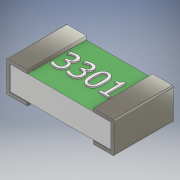
# Autodesk Inventor part: 21-1001
Saved by Autodesk Inventor 2018 (Build 220112000, 112)
## iProperties
Created: 2019-09-21
Part Number: 21-1001
Material: Copper
Document SubType Name: Modeling
Designer: Bradley
Density: 8.94 g/cm^3
Appearance: Smooth - White
Author: Bradley
Autodesk Inventor part; units mm, degrees
ref_plane "YZ Plane" through (0, 0, 0) normal (1, 0, 0) x (0, 1, 0)
ref_plane "XZ Plane" through (0, 0, 0) normal (0, 1, 0) x (-1, 0, 0)
ref_plane "XY Plane" through (0, 0, 0) normal (0, 0, 1) x (1, 0, 0)
sketch "Sketch1" plane through (0, 0, 0) normal (0, 1, 0) x (-1, 0, 0)
  line L0 (0.725, 0.175) -> (-0.725, 0.175)
  line L1 (-0.725, 0.175) -> (-0.725, -0.175)
  line L2 (-0.725, -0.175) -> (0.725, -0.175)
  line L3 (0.725, -0.175) -> (0.725, 0.175)
  line L4 (0.475, 0.175) -> (0.475, 0.225)
  line L5 (0.475, 0.225) -> (0.775, 0.225)
  line L6 (0.775, 0.225) -> (0.775, -0.225)
  line L7 (0.775, -0.225) -> (0.475, -0.225)
  line L8 (0.475, -0.225) -> (0.475, -0.175)
  line L9 (-0.475, 0.175) -> (-0.475, 0.225)
  line L10 (-0.475, 0.225) -> (-0.775, 0.225)
  line L11 (-0.775, 0.225) -> (-0.775, -0.225)
  line L12 (-0.775, -0.225) -> (-0.475, -0.225)
  line L13 (-0.475, -0.175) -> (-0.475, -0.225)
  line L14 (0.475, 0.175) -> (-0.475, 0.175)
  point P0 (0, 0)
  point P1 (0, 0.175)
  point P2 (0.725, 0)
  dimension "d0" = 1.55
  dimension "d1" = 0.05
  dimension "d2" = 0.05
  dimension "d3" = 0.45
  dimension "d4" = 0.3
  constraints: 30 end point, 12 point on line, 7 perpendicular, 3 collinear, 3 midpoint, 2 parallel, 1 horizontal, 1 horizontal alignment, 1 vertical, 1 vertical alignment
  measures "d0" distance between parallel lines of L11 L6
  measures "d1" distance of L7.end L8.end
  measures "d2" distance between parallel lines of L6 L3
  measures "d3" distance of L5.end L6.end
  measures "d4" distance of L6.end L7.end
extrude "Extrusion1" add sketch "Sketch1" along normal mid plane 0.85 contours L0 L4 L5 L6 L7 L8 L2 L3 | L0 L1 L2 L13 L12 L11 L10 L9
extrude "Extrusion2" add sketch "Sketch1" along normal mid plane 0.84 contours L3 L2 L1 L0
sketch "Sketch2" plane through (-0.475, -0.42, 0.175) normal (0, 0, 1) x (1, 0, 0)
  line L0 (0, 0) -> (0, 0.84) projected
  line L1 (0.95, 0) -> (0, 0) projected
  line L2 (0.95, 0) -> (0.95, 0.84) projected
  line L3 (0, 0.84) -> (0.95, 0.84) projected
  line L4 (0, 0.42) -> (0.95, 0.42) construction
  spline S0 degree 2 poles (0.1276, 0.5416) (0.1167, 0.5416) (0.095, 0.5362) (0.0846, 0.5321) knots 0 0 0 1 2 2 2
  spline S1 degree 2 poles (0.0846, 0.5321) (0.0748, 0.5279) (0.0605, 0.5192) (0.0549, 0.5153) knots 0 0 0 1 2 2 2
  line L5 (0.0549, 0.5153) -> (0.0525, 0.5153)
  line L6 (0.0525, 0.5153) -> (0.0525, 0.5578)
  spline S2 degree 2 poles (0.0525, 0.5578) (0.0656, 0.5649) (0.1106, 0.5763) (0.1308, 0.5763) knots 0 0 0 1 2 2 2
  spline S3 degree 2 poles (0.1308, 0.5763) (0.1512, 0.5763) (0.1816, 0.5681) (0.194, 0.5593) knots 0 0 0 1 2 2 2
  spline S4 degree 2 poles (0.194, 0.5593) (0.2071, 0.5498) (0.2207, 0.5224) (0.2207, 0.5039) knots 0 0 0 1 2 2 2
  spline S5 degree 2 poles (0.2207, 0.5039) (0.2207, 0.4791) (0.1881, 0.4416) (0.1653, 0.4368) knots 0 0 0 1 2 2 2
  line L7 (0.1653, 0.4368) -> (0.1653, 0.4339)
  spline S6 degree 2 poles (0.1653, 0.4339) (0.1748, 0.4319) (0.1964, 0.4232) (0.2056, 0.4144) knots 0 0 0 1 2 2 2
  spline S7 degree 2 poles (0.2056, 0.4144) (0.2149, 0.4059) (0.2265, 0.3787) (0.2265, 0.359) knots 0 0 0 1 2 2 2
  spline S8 degree 2 poles (0.2265, 0.359) (0.2265, 0.3388) (0.2127, 0.3045) (0.2, 0.2914) knots 0 0 0 1 2 2 2
  spline S9 degree 2 poles (0.2, 0.2914) (0.1869, 0.2778) (0.1497, 0.2637) (0.1261, 0.2637) knots 0 0 0 1 2 2 2
  spline S10 degree 2 poles (0.1261, 0.2637) (0.1035, 0.2637) (0.0593, 0.2746) (0.0442, 0.2822) knots 0 0 0 1 2 2 2
  line L8 (0.0442, 0.2822) -> (0.0442, 0.3247)
  line L9 (0.0442, 0.3247) -> (0.0471, 0.3247)
  spline S11 degree 2 poles (0.0471, 0.3247) (0.0598, 0.3155) (0.1026, 0.2984) (0.1237, 0.2984) knots 0 0 0 1 2 2 2
  spline S12 degree 2 poles (0.1237, 0.2984) (0.1361, 0.2984) (0.1609, 0.3062) (0.1692, 0.3152) knots 0 0 0 1 2 2 2
  spline S13 degree 2 poles (0.1692, 0.3152) (0.1772, 0.3242) (0.1857, 0.3456) (0.1857, 0.3619) knots 0 0 0 1 2 2 2
  spline S14 degree 2 poles (0.1857, 0.3619) (0.1857, 0.3782) (0.1762, 0.3993) (0.1677, 0.4054) knots 0 0 0 1 2 2 2
  spline S15 degree 2 poles (0.1677, 0.4054) (0.1592, 0.4115) (0.1361, 0.4161) (0.1225, 0.4161) knots 0 0 0 1 2 2 2
  line L10 (0.1225, 0.4161) -> (0.1055, 0.4161)
  line L11 (0.1055, 0.4161) -> (0.1055, 0.4494)
  line L12 (0.1055, 0.4494) -> (0.1188, 0.4494)
  spline S16 degree 2 poles (0.1188, 0.4494) (0.1458, 0.4494) (0.1799, 0.4752) (0.1799, 0.4997) knots 0 0 0 1 2 2 2
  spline S17 degree 2 poles (0.1799, 0.4997) (0.1799, 0.5112) (0.1711, 0.5275) (0.1641, 0.5323) knots 0 0 0 1 2 2 2
  spline S18 degree 2 poles (0.1641, 0.5323) (0.1565, 0.5374) (0.138, 0.5416) (0.1276, 0.5416) knots 0 0 0 1 2 2 2
  spline S19 degree 2 poles (0.3527, 0.5416) (0.3418, 0.5416) (0.3201, 0.5362) (0.3097, 0.5321) knots 0 0 0 1 2 2 2
  spline S20 degree 2 poles (0.3097, 0.5321) (0.3, 0.5279) (0.2856, 0.5192) (0.28, 0.5153) knots 0 0 0 1 2 2 2
  line L13 (0.28, 0.5153) -> (0.2776, 0.5153)
  line L14 (0.2776, 0.5153) -> (0.2776, 0.5578)
  spline S21 degree 2 poles (0.2776, 0.5578) (0.2907, 0.5649) (0.3357, 0.5763) (0.3559, 0.5763) knots 0 0 0 1 2 2 2
  spline S22 degree 2 poles (0.3559, 0.5763) (0.3763, 0.5763) (0.4067, 0.5681) (0.4191, 0.5593) knots 0 0 0 1 2 2 2
  spline S23 degree 2 poles (0.4191, 0.5593) (0.4322, 0.5498) (0.4458, 0.5224) (0.4458, 0.5039) knots 0 0 0 1 2 2 2
  spline S24 degree 2 poles (0.4458, 0.5039) (0.4458, 0.4791) (0.4132, 0.4416) (0.3904, 0.4368) knots 0 0 0 1 2 2 2
  line L15 (0.3904, 0.4368) -> (0.3904, 0.4339)
  spline S25 degree 2 poles (0.3904, 0.4339) (0.3999, 0.4319) (0.4215, 0.4232) (0.4308, 0.4144) knots 0 0 0 1 2 2 2
  spline S26 degree 2 poles (0.4308, 0.4144) (0.44, 0.4059) (0.4517, 0.3787) (0.4517, 0.359) knots 0 0 0 1 2 2 2
  spline S27 degree 2 poles (0.4517, 0.359) (0.4517, 0.3388) (0.4378, 0.3045) (0.4252, 0.2914) knots 0 0 0 1 2 2 2
  spline S28 degree 2 poles (0.4252, 0.2914) (0.412, 0.2778) (0.3748, 0.2637) (0.3513, 0.2637) knots 0 0 0 1 2 2 2
  spline S29 degree 2 poles (0.3513, 0.2637) (0.3286, 0.2637) (0.2844, 0.2746) (0.2693, 0.2822) knots 0 0 0 1 2 2 2
  line L16 (0.2693, 0.2822) -> (0.2693, 0.3247)
  line L17 (0.2693, 0.3247) -> (0.2722, 0.3247)
  spline S30 degree 2 poles (0.2722, 0.3247) (0.2849, 0.3155) (0.3277, 0.2984) (0.3488, 0.2984) knots 0 0 0 1 2 2 2
  spline S31 degree 2 poles (0.3488, 0.2984) (0.3612, 0.2984) (0.386, 0.3062) (0.3943, 0.3152) knots 0 0 0 1 2 2 2
  spline S32 degree 2 poles (0.3943, 0.3152) (0.4023, 0.3242) (0.4108, 0.3456) (0.4108, 0.3619) knots 0 0 0 1 2 2 2
  spline S33 degree 2 poles (0.4108, 0.3619) (0.4108, 0.3782) (0.4013, 0.3993) (0.3928, 0.4054) knots 0 0 0 1 2 2 2
  spline S34 degree 2 poles (0.3928, 0.4054) (0.3843, 0.4115) (0.3612, 0.4161) (0.3476, 0.4161) knots 0 0 0 1 2 2 2
  line L18 (0.3476, 0.4161) -> (0.3306, 0.4161)
  line L19 (0.3306, 0.4161) -> (0.3306, 0.4494)
  line L20 (0.3306, 0.4494) -> (0.344, 0.4494)
  spline S35 degree 2 poles (0.344, 0.4494) (0.3709, 0.4494) (0.405, 0.4752) (0.405, 0.4997) knots 0 0 0 1 2 2 2
  spline S36 degree 2 poles (0.405, 0.4997) (0.405, 0.5112) (0.3962, 0.5275) (0.3892, 0.5323) knots 0 0 0 1 2 2 2
  spline S37 degree 2 poles (0.3892, 0.5323) (0.3816, 0.5374) (0.3632, 0.5416) (0.3527, 0.5416) knots 0 0 0 1 2 2 2
  spline S38 degree 2 poles (0.6836, 0.42) (0.6836, 0.3393) (0.6367, 0.2637) (0.5878, 0.2637) knots 0 0 0 1 2 2 2
  spline S39 degree 2 poles (0.5878, 0.2637) (0.5382, 0.2637) (0.4918, 0.3407) (0.4918, 0.4198) knots 0 0 0 1 2 2 2
  spline S40 degree 2 poles (0.4918, 0.4198) (0.4918, 0.501) (0.5387, 0.5761) (0.5878, 0.5761) knots 0 0 0 1 2 2 2
  spline S41 degree 2 poles (0.5878, 0.5761) (0.6372, 0.5761) (0.6836, 0.4983) (0.6836, 0.42) knots 0 0 0 1 2 2 2
  spline S42 degree 2 poles (0.6321, 0.3286) (0.6379, 0.3434) (0.6427, 0.3891) (0.6427, 0.42) knots 0 0 0 1 2 2 2
  spline S43 degree 2 poles (0.6427, 0.42) (0.6427, 0.4509) (0.6379, 0.4963) (0.6318, 0.5117) knots 0 0 0 1 2 2 2
  spline S44 degree 2 poles (0.6318, 0.5117) (0.6257, 0.527) (0.6046, 0.5428) (0.5878, 0.5428) knots 0 0 0 1 2 2 2
  spline S45 degree 2 poles (0.5878, 0.5428) (0.571, 0.5428) (0.5494, 0.527) (0.5431, 0.5112) knots 0 0 0 1 2 2 2
  spline S46 degree 2 poles (0.5431, 0.5112) (0.537, 0.4959) (0.5326, 0.4492) (0.5326, 0.4198) knots 0 0 0 1 2 2 2
  spline S47 degree 2 poles (0.5326, 0.4198) (0.5326, 0.3882) (0.5365, 0.3459) (0.5428, 0.3293) knots 0 0 0 1 2 2 2
  spline S48 degree 2 poles (0.5428, 0.3293) (0.5487, 0.3138) (0.5703, 0.297) (0.5878, 0.297) knots 0 0 0 1 2 2 2
  spline S49 degree 2 poles (0.5878, 0.297) (0.6043, 0.297) (0.626, 0.3128) (0.6321, 0.3286) knots 0 0 0 1 2 2 2
  line L21 (0.8919, 0.27) -> (0.7456, 0.27)
  line L22 (0.7456, 0.27) -> (0.7456, 0.3006)
  line L23 (0.7456, 0.3006) -> (0.8, 0.3006)
  line L24 (0.8, 0.3006) -> (0.8, 0.5017)
  line L25 (0.8, 0.5017) -> (0.7456, 0.5017)
  line L26 (0.7456, 0.5017) -> (0.7456, 0.5292)
  spline S50 degree 2 poles (0.7456, 0.5292) (0.7765, 0.5292) (0.8056, 0.5467) (0.8076, 0.571) knots 0 0 0 1 2 2 2
  line L27 (0.8076, 0.571) -> (0.8387, 0.571)
  line L28 (0.8387, 0.571) -> (0.8387, 0.3006)
  line L29 (0.8387, 0.3006) -> (0.8919, 0.3006)
  line L30 (0.8919, 0.3006) -> (0.8919, 0.27)
  point P0 (0.475, 0.42)
  constraints: 2 end point, 2 midpoint, 1 horizontal
extrude "Extrusion3" add sketch "Sketch2" along normal blind 0.02 contours S0 S1 L5 L6 S2 S3 S4 S5 L7 S6 S7 S8 S9 S10 L8 L9 S11 S12 S13 S14 S15 L10 L11 L12 S16 S17 S18 | S19 S20 L13 L14 S21 S22 S23 S24 L15 S25 S26 S27 S28 S29 L16 L17 S30 S31 S32 S33 S34 L18 L19 L20 S35 S36 S37 | S38 S39 S40 S41 | L21 L22 L23 L24 L25 L26 S50 L27 L28 L29 L30
fillet "Fillet1" radius 0.02 4 edges at (-0.775, 0, 0.225) (-0.775, 0, -0.225) (0.775, 0, 0.225) (0.775, 0, -0.225)
equation "\"d2\" = d1"
body "Solid1"
